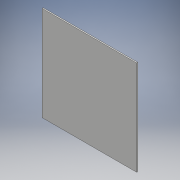
# Autodesk Inventor part: solar
Saved by Autodesk Inventor 2017 (Build 210142000, 142)
## iProperties
Created: 2019-04-28
Part Number: solar
Material: Generic
Document SubType Name: Modeling
Designer: simulator
Density: 1 g/cm^3
Appearance: Default
Author: simulator
Autodesk Inventor part; units mm, degrees
ref_plane "YZ Plane" through (0, 0, 0) normal (1, 0, 0) x (0, 1, 0)
ref_plane "XZ Plane" through (0, 0, 0) normal (0, 1, 0) x (-1, 0, 0)
ref_plane "XY Plane" through (0, 0, 0) normal (0, 0, 1) x (1, 0, 0)
sketch "Sketch1" plane through (0, 0, 0) normal (0, 1, 0) x (-1, 0, 0)
  line L0 (-82.5, 82.5) -> (82.5, 82.5)
  line L1 (82.5, 82.5) -> (82.5, -82.5)
  line L2 (82.5, -82.5) -> (-82.5, -82.5)
  line L3 (-82.5, -82.5) -> (-82.5, 82.5)
  line L4 (-82.5, 82.5) -> (82.5, -82.5) construction
  line L5 (82.5, 82.5) -> (-82.5, -82.5) construction
  point P0 (0, 0)
  dimension "d0" = 165
  dimension "d1" = 165
  constraints: 12 end point, 2 midpoint, 2 parallel, 1 horizontal, 1 perpendicular
  measures "d0" distance of L1.end L2.end
  measures "d1" distance of L0.end L1.end
extrude "Extrusion1" add sketch "Sketch1" along normal blind 2
body "Solid1"
